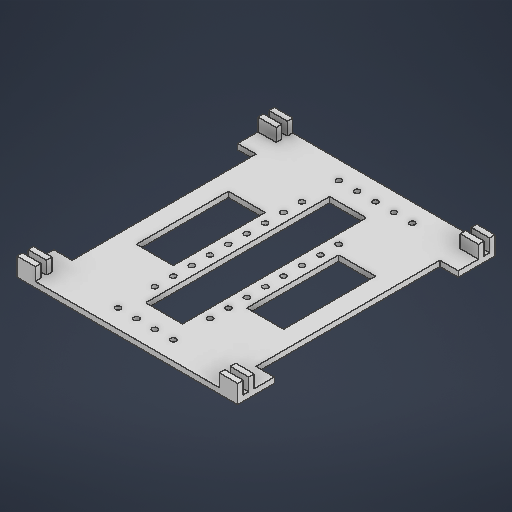
# Autodesk Inventor part: base_2
Saved by Autodesk Inventor 2026.1 (Build 301233000, 233)
## iProperties
Created: 2025-10-15
Part Number: base_2
Material: Generic
Document SubType Name: Modeling
Designer: emanuel
Density: 1 g/cm^3
Appearance: Default
Author: emanuel
Autodesk Inventor part; units mm, degrees
ref_plane "YZ Plane" through (0, 0, 0) normal (1, 0, 0) x (0, 1, 0)
ref_plane "XZ Plane" through (0, 0, 0) normal (0, 1, 0) x (-1, 0, 0)
ref_plane "XY Plane" through (0, 0, 0) normal (0, 0, 1) x (1, 0, 0)
sketch "Sketch2" plane through (0, 0, 0) normal (0, 1, 0) x (-1, 0, 0)
  line L0 (0, 0) -> (120, 0)
  line L1 (120, 0) -> (120, -140)
  line L2 (120, -140) -> (0, -140)
  line L3 (0, -140) -> (0, 0)
  line L4 (120, 0) -> (0, 0)
  line L5 (0, 0) -> (0, -20)
  line L6 (0, -20) -> (120, -20)
  line L7 (120, -20) -> (120, 0)
  line L8 (120, -140) -> (0, -140)
  line L9 (0, -140) -> (0, -120)
  line L10 (0, -120) -> (120, -120)
  line L11 (120, -120) -> (120, -140)
  line L12 (120, -20) -> (110, -20)
  line L13 (110, -20) -> (110, -120)
  line L14 (110, -120) -> (120, -120)
  line L15 (120, -120) -> (120, -20)
  line L16 (110, -20) -> (70, -20)
  line L17 (70, -20) -> (70, -120)
  line L18 (70, -120) -> (110, -120)
  line L19 (110, -120) -> (110, -20)
  line L20 (0, -20) -> (10, -20)
  line L21 (10, -20) -> (10, -120)
  line L22 (10, -120) -> (0, -120)
  line L23 (0, -120) -> (0, -20)
  line L24 (70, -20) -> (10, -20)
  line L25 (10, -20) -> (10, -120)
  line L26 (10, -120) -> (70, -120)
  line L27 (70, -120) -> (70, -20)
  line L28 (70, -20) -> (90, -20)
  line L29 (90, -120) -> (70, -120)
  line L30 (70, -120) -> (70, -20)
  line L31 (10, -20) -> (40, -20)
  line L32 (40, -120) -> (10, -120)
  line L33 (10, -120) -> (10, -20)
  line L34 (10, -20) -> (50, -20)
  line L35 (50, -20) -> (50, -120)
  line L36 (50, -120) -> (10, -120)
  line L37 (10, -120) -> (10, -20)
  line L38 (120, -10) -> (0, -10)
  line L39 (120, -10) -> (85, -10)
  line L40 (0, -10) -> (35, -10)
  line L41 (120, -130) -> (0, -130)
  line L42 (120, -130) -> (85, -130)
  line L43 (85, -10) -> (75, -10)
  line L44 (75, -10) -> (65, -10)
  line L45 (65, -10) -> (55, -10)
  line L46 (55, -10) -> (45, -10)
  line L47 (45, -10) -> (35, -10)
  circle A0 centre (45, -10) radius 1.5
  circle A1 centre (55, -10) radius 1.5
  circle A2 centre (65, -10) radius 1.5
  circle A3 centre (75, -10) radius 1.5
  line L48 (85, -130) -> (75, -130)
  line L49 (75, -130) -> (65, -130)
  line L50 (65, -130) -> (55, -130)
  line L51 (55, -130) -> (45, -130)
  line L52 (45, -130) -> (35, -130)
  circle A4 centre (75, -130) radius 1.5
  circle A5 centre (65, -130) radius 1.5
  circle A6 centre (55, -130) radius 1.5
  circle A7 centre (45, -130) radius 1.5
  circle A8 centre (35, -130) radius 1.5
  line L53 (110, -120) -> (90, -120)
  line L54 (90, -120) -> (90, -70)
  line L55 (90, -70) -> (110, -70)
  line L56 (110, -70) -> (110, -120)
  line L57 (50, -20) -> (30, -20)
  line L58 (30, -20) -> (30, -70)
  line L59 (30, -70) -> (50, -70)
  line L60 (50, -70) -> (50, -20)
  line L61 (100, -45) -> (80, -45)
  line L62 (80, -45) -> (80, -95)
  line L63 (80, -95) -> (100, -95)
  line L64 (100, -95) -> (100, -45)
  line L65 (100, -45) -> (80, -95) construction
  line L66 (80, -45) -> (100, -95) construction
  line L67 (40, -45) -> (20, -45)
  line L68 (20, -45) -> (20, -95)
  line L69 (20, -95) -> (40, -95)
  line L70 (40, -95) -> (40, -45)
  line L71 (40, -45) -> (20, -95) construction
  line L72 (20, -45) -> (40, -95) construction
  dimension "d0" = 120
  dimension "d1" = 140
  dimension "d2" = 20
  dimension "d3" = 20
  dimension "d4" = 10
  dimension "d5" = 40
  dimension "d6" = 10
  dimension "d7" = 40
  dimension "d10" = 35
  dimension "d11" = 35
  dimension "d12" = 35
  dimension "d13" = 10
  dimension "d14" = 10
  dimension "d15" = 10
  dimension "d16" = 10
  dimension "d17" = 10
  dimension "d18" = 3
  dimension "d19" = 3
  dimension "d20" = 3
  dimension "d21" = 3
  dimension "d22" = 10
  dimension "d23" = 10
  dimension "d24" = 10
  dimension "d25" = 10
  dimension "d26" = 10
  dimension "d27" = 3
  dimension "d28" = 3
  dimension "d29" = 3
  dimension "d30" = 3
  dimension "d31" = 3
  dimension "d32" = 20
  dimension "d33" = 50
  dimension "d34" = 20
  dimension "d35" = 50
  dimension "d36" = 20
  dimension "d37" = 50
  dimension "d38" = 20
  dimension "d39" = 50
  constraints: 146 end point, 27 equal length, 18 point on line, 14 horizontal, 12 perpendicular, 10 midpoint, 9 centre point, 9 coincident
  measures "d0" distance of L1.end L2.end
  measures "d1" distance of L0.end L1.end
  measures "d2" distance of L5.end L4.end
  measures "d3" distance of L8.end L9.end
  measures "d4" distance of L14.end L13.end
  measures "d5" distance of L18.end L17.end
  measures "d6" distance of L21.end L22.end
  measures "d7" distance of L35.end L36.end
  measures "d10" distance of L38.start L39.end
  measures "d11" distance of L38.end L40.end
  measures "d12" distance of L41.start L42.end
  measures "d13" distance of L39.end L43.end
  measures "d14" distance of L43.end L44.end
  measures "d15" distance of L44.end L45.end
  measures "d16" distance of L45.end L46.end
  measures "d17" distance of L46.end L40.end
  measures "d18" diameter of A0
  measures "d19" diameter of A1
  measures "d20" diameter of A2
  measures "d21" diameter of A3
  measures "d22" distance of L42.end L48.end
  measures "d23" distance of L48.end L49.end
  measures "d24" distance of L49.end L50.end
  measures "d25" distance of L50.end L51.end
  measures "d26" distance of L51.end L52.end
  measures "d27" diameter of A4
  measures "d28" diameter of A5
  measures "d29" diameter of A6
  measures "d30" diameter of A7
  measures "d31" diameter of A8
  measures "d32" distance of L54.end L55.end
  measures "d33" distance of L53.end L54.end
  measures "d34" distance of L59.end L58.end
  measures "d35" distance of L58.end L57.end
  measures "d36" distance of L63.end L62.end
  measures "d37" distance of L62.end L61.end
  measures "d38" distance of L69.end L68.end
  measures "d39" distance of L68.end L67.end
extrude "Extrusion1" add sketch "Sketch2" along normal blind 3 contours L0 L1 L38 A3 A2 A1 A0 L3 | L38 A0 A1 A2 A3 L1 L6 L3 | L10 L1 L41 A4 A5 A6 A7 A8 L3 | L6 L58 L67 L68 L69 L70 L59 L35 L10 L21 | L13 L55 L64 L61 L62 L63 L54 L10 L17 L6 | L41 A8 A7 A6 A5 A4 L1 L2 L3 | L6 L35 L59 L70 L67 L58 | L10 L54 L63 L64 L55 L13
sketch "Sketch3" plane through (0, 3, 0) normal (0, 1, 0) x (1, 0, 0)
  line L0 (-40, 45) -> (-40, 95) projected
  line L1 (-50, 120) -> (-40, 120)
  line L2 (-40, 120) -> (-40, 45)
  line L3 (-40, 45) -> (-50, 45)
  line L4 (-50, 45) -> (-50, 120)
  line L5 (-50, 20) -> (-70, 20) projected
  line L6 (-50, 20) -> (-40, 20)
  line L7 (-40, 20) -> (-40, 120)
  line L8 (-40, 120) -> (-50, 120)
  line L9 (-50, 120) -> (-50, 20)
  line L10 (-70, 20) -> (-70, 120) projected
  line L11 (-80, 95) -> (-80, 45) projected
  line L12 (-70, 120) -> (-80, 120)
  line L13 (-80, 120) -> (-80, 45)
  line L14 (-80, 45) -> (-70, 45)
  line L15 (-70, 45) -> (-70, 120)
  line L16 (-80, 120) -> (-70, 120)
  line L17 (-70, 120) -> (-70, 20)
  line L18 (-70, 20) -> (-80, 20)
  line L19 (-80, 20) -> (-80, 120)
  line L20 (-75, 120) -> (-75, 20)
  line L21 (-45, 120) -> (-45, 20)
  line L22 (-75, 120) -> (-75, 110)
  line L23 (-75, 110) -> (-75, 100)
  line L24 (-75, 100) -> (-75, 90)
  line L25 (-75, 90) -> (-75, 80)
  line L26 (-75, 80) -> (-75, 70)
  line L27 (-75, 70) -> (-75, 60)
  line L28 (-75, 60) -> (-75, 50)
  line L29 (-75, 50) -> (-75, 40)
  line L30 (-75, 40) -> (-75, 20)
  line L31 (-75, 40) -> (-75, 30)
  line L32 (-45, 120) -> (-45, 110)
  line L33 (-45, 110) -> (-45, 100)
  line L34 (-45, 100) -> (-45, 90)
  line L35 (-45, 90) -> (-45, 80)
  line L36 (-45, 80) -> (-45, 70)
  line L37 (-45, 70) -> (-45, 60)
  line L38 (-45, 60) -> (-45, 50)
  line L39 (-45, 50) -> (-45, 40)
  line L40 (-45, 40) -> (-45, 30)
  line L41 (-45, 30) -> (-45, 20)
  circle A0 centre (-75, 110) radius 1.5
  circle A1 centre (-75, 100) radius 1.5
  circle A2 centre (-75, 90) radius 1.5
  circle A3 centre (-75, 80) radius 1.5
  circle A4 centre (-75, 70) radius 1.5
  circle A5 centre (-75, 60) radius 1.5
  circle A6 centre (-75, 50) radius 1.5
  circle A7 centre (-75, 40) radius 1.5
  circle A8 centre (-75, 30) radius 1.5
  circle A9 centre (-45, 110) radius 1.5
  circle A10 centre (-45, 100) radius 1.5
  circle A11 centre (-45, 90) radius 1.5
  circle A12 centre (-45, 80) radius 1.5
  circle A13 centre (-45, 70) radius 1.5
  circle A14 centre (-45, 60) radius 1.5
  circle A15 centre (-45, 50) radius 1.5
  circle A16 centre (-45, 40) radius 1.5
  circle A17 centre (-45, 30) radius 1.5
  point P0 (0, 0)
  dimension "d40" = 10
  dimension "d41" = 10
  dimension "d42" = 10
  dimension "d43" = 10
  dimension "d44" = 10
  dimension "d45" = 10
  dimension "d46" = 10
  dimension "d47" = 10
  dimension "d48" = 20
  dimension "d49" = 10
  dimension "d50" = 10
  dimension "d51" = 10
  dimension "d52" = 10
  dimension "d53" = 10
  dimension "d54" = 10
  dimension "d55" = 10
  dimension "d56" = 10
  dimension "d57" = 10
  dimension "d58" = 10
  dimension "d59" = 3
  dimension "d60" = 3
  constraints: 72 end point, 18 centre point, 18 coincident, 8 parallel, 5 midpoint, 4 horizontal, 4 perpendicular, 2 collinear, 23 other
  measures "d40" distance of L22.start L22.end
  measures "d41" distance of L22.end L23.end
  measures "d42" distance of L23.end L24.end
  measures "d43" distance of L24.end L25.end
  measures "d44" distance of L25.end L26.end
  measures "d45" distance of L26.end L27.end
  measures "d46" distance of L27.end L28.end
  measures "d47" distance of L28.end L29.end
  measures "d48" distance of L29.end L30.end
  measures "d49" distance of L32.start L32.end
  measures "d50" distance of L32.end L33.end
  measures "d51" distance of L33.end L34.end
  measures "d52" distance of L34.end L35.end
  measures "d53" distance of L35.end L36.end
  measures "d54" distance of L36.end L37.end
  measures "d55" distance of L37.end L38.end
  measures "d56" distance of L38.end L39.end
  measures "d57" distance of L39.end L40.end
  measures "d58" distance of L40.end L41.end
  measures "d59" diameter of A0
  measures "d60" diameter of A9
extrude "Extrusion2" cut sketch "Sketch3" against normal up to surface (3 mm away) contours A15 L21 | L21 A15 | A16 L21 | L21 A16 | A17 L21 | L21 A17 | A14 L21 | L21 A14 | A10 L21 | L21 A10 | A13 L21 | L21 A13 | A11 L21 | L21 A11 | A12 L21 | L21 A12 | A8 L20 | L20 A8 | A6 L20 | L20 A6 | A7 L20 | L20 A7 | A0 L20 | L20 A0 | A5 L20 | L20 A5 | A1 L20 | L20 A1 | A4 L20 | L20 A4 | A2 L20 | L20 A2 | A3 L20 | L20 A3
sketch "Sketch4" plane through (0, 3, 0) normal (0, 1, 0) x (1, 0, 0)
  line L0 (0, 140) -> (-120, 140) projected
  line L1 (0, 120) -> (0, 140) projected
  line L2 (-120, 140) -> (0, 140)
  line L3 (0, 140) -> (0, 137)
  line L4 (0, 137) -> (-120, 137)
  line L5 (-120, 137) -> (-120, 140)
  line L6 (-120, 137) -> (0, 137)
  line L7 (0, 137) -> (0, 134)
  line L8 (0, 134) -> (-120, 134)
  line L9 (-120, 134) -> (-120, 137)
  line L10 (-120, 134) -> (0, 134)
  line L11 (0, 134) -> (0, 131)
  line L12 (0, 131) -> (-120, 131)
  line L13 (-120, 131) -> (-120, 134)
  line L14 (-120, 0) -> (0, 0) projected
  line L15 (-120, 0) -> (0, 0)
  line L16 (0, 0) -> (0, 6)
  line L17 (0, 6) -> (-120, 6)
  line L18 (-120, 6) -> (-120, 0)
  line L19 (-120, 6) -> (0, 6)
  line L20 (0, 6) -> (0, 3)
  line L21 (0, 3) -> (-120, 3)
  line L22 (-120, 3) -> (-120, 6)
  line L23 (0, 3) -> (-120, 3)
  line L24 (-120, 3) -> (-120, 9)
  line L25 (-120, 9) -> (0, 9)
  line L26 (0, 9) -> (0, 3)
  line L27 (-120, 140) -> (-110, 140)
  line L28 (-110, 140) -> (-110, 0)
  line L29 (-110, 0) -> (-120, 0)
  line L30 (-120, 0) -> (-120, 140)
  line L31 (0, 140) -> (-10, 140)
  line L32 (-10, 140) -> (-10, 0)
  line L33 (-10, 0) -> (0, 0)
  line L34 (0, 0) -> (0, 140)
  line L35 (-10, 0) -> (0, 0)
  line L36 (0, 0) -> (0, 3)
  line L37 (0, 3) -> (-10, 3)
  line L38 (-10, 3) -> (-10, 0)
  point P0 (-10, 134)
  point P1 (-10, 131)
  point P2 (-10, 137)
  point P3 (-110, 131)
  point P4 (-110, 134)
  point P5 (-110, 137)
  point P6 (-110, 6)
  point P7 (-110, 9)
  point P8 (-110, 0)
  point P9 (-110, 3)
  point P10 (-10, 9)
  point P11 (-10, 6)
  point P12 (-10, 3)
  point P13 (-10, 0)
  dimension "d63" = 3
  dimension "d64" = 120
  dimension "d65" = 3
  dimension "d66" = 3
  dimension "d67" = 6
  dimension "d68" = 6
  dimension "d69" = 10
  dimension "d70" = 10
  constraints: 72 end point, 18 parallel, 9 horizontal, 9 perpendicular, 6 point on line, 1 midpoint
  measures "d63" distance of L2.end L3.end
  measures "d64" distance of L7.end L8.end
  measures "d65" distance of L6.end L7.end
  measures "d66" distance of L10.end L11.end
  measures "d67" distance of L16.end L15.end
  measures "d68" distance of L23.end L24.end
  measures "d69" distance of L28.end L29.end
  measures "d70" distance of L33.end L32.end
extrude "Extrusion3" add sketch "Sketch4" along normal blind 7 contours L1 L4 L32 L0 | L28 L4 L5 L0 | L1 L12 L32 L8 | L28 L12 L13 L8 | L25 L26 L17 L32 | L28 L17 L24 L25 | L21 L16 L14 L32 | L28 L14 L18 L21
equation "\"d8\" = d21"
equation "\"d61\" = d21"
body "Solid1"
